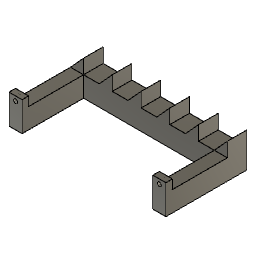
Back_gripper_assembly v17 (Autodesk Fusion 360 archive; units mm, degrees)
design "Wall_reverse"
Autodesk Fusion 360 part; units mm, degrees
sketch "Sketch1" plane through (0, 0, 0) normal (0, 0, 1) x (1, 0, 0)
  line L0 (30, -7.5) -> (-30, -7.5)
  line L1 (-30, -7.5) -> (-30, 7.5)
  line L2 (-30, 7.5) -> (30, 7.5)
  line L3 (30, 7.5) -> (30, -7.5)
  line L4 (30, -7.5) -> (-30, 7.5) construction
  line L5 (-30, -7.5) -> (30, 7.5) construction
  dimension "d1" = 60
  dimension "d2" = 15
  constraint horizontal L0
  constraint perpendicular L0 L1
  constraint parallel L0 L2
  constraint parallel L1 L3
  constraint coincident L4 origin
  constraint coincident L5 origin
  measures "d1" distance of L1.end L2.end
  measures "d2" distance of L0.end L1.end
extrude "Extrude1" add sketch "Sketch1" along normal blind 15.5 makes body 1
sketch "Sketch2" plane through (0, 0, 15.5) normal (0, 0, 1) x (-1, 0, 0)
  line L0 (-30, -7.5) -> (30, -7.5)
  line L1 (30, -7.5) -> (30, 7.5)
  line L2 (30, 7.5) -> (-30, 7.5)
  line L3 (-30, 7.5) -> (-30, -7.5)
  line L4 (-30, -7.5) -> (-15, -7.5)
  line L5 (-15, -7.5) -> (-15, 12.5)
  line L6 (-15, 12.5) -> (-30, 12.5)
  line L7 (-30, 12.5) -> (-30, -7.5)
  dimension "d5" = 15
  dimension "d6" = 20
  constraint horizontal L4
  constraint vertical L5
  constraint horizontal L6
  constraint vertical L7
  constraint coincident L0.start L3.end
  measures "d5" distance of L0.start L4.end
  measures "d6" distance of L0.start L6.end
sketch "Sketch3" plane through (0, -7.5, 0) normal (0, -1, 0) x (1, 0, 0)
  line L0 (-30, 0) -> (30, 0)
  line L1 (30, 0) -> (30, 15.5)
  line L2 (30, 15.5) -> (-30, 15.5)
  line L3 (-30, 15.5) -> (-30, 0)
  line L4 (20, 15.5) -> (30, 15.5)
  line L5 (30, 15.5) -> (30, 0)
  line L6 (30, 0) -> (20, 0)
  line L7 (20, 0) -> (20, 15.5)
  constraint horizontal L4
  constraint vertical L5
  constraint horizontal L6
  constraint vertical L7
  constraint coincident L0.end L1.start
  constraint coincident L1.end L2.start
extrude "Extrude3" add sketch "Sketch3" along normal blind 47 contours L0 L1 L2 L4 L5 L6 L7 bodies 1
sketch "Sketch4" plane through (0, 0, 15.5) normal (0, 0, 1) x (-1, 0, 0)
  line L0 (-30, 54.5) -> (-30, -7.5)
  line L1 (-20, 7.5) -> (-20, 54.5)
  line L2 (-20, 54.5) -> (-30, 54.5)
  line L3 (-20, 54.5) -> (-61.6412, 54.5)
  line L4 (-61.6412, 54.5) -> (-61.6412, 49.5)
  line L5 (-61.6412, 49.5) -> (-20, 49.5)
  line L6 (-20, 49.5) -> (-20, 54.5)
  line L7 (-30, -7.5) -> (30, -7.5)
  line L8 (30, -7.5) -> (30, 7.5)
  line L9 (30, 7.5) -> (-20, 7.5)
  dimension "d11" = 5
  constraint horizontal L3
  constraint vertical L4
  constraint horizontal L5
  constraint vertical L6
  constraint coincident L1.end L2.start
  measures "d11" distance of L1.end L5.end
extrude "Extrude4" add sketch "Sketch4" along normal blind 7 contours L0 L1 L2 L3 L5 L6 bodies 1
mirror "Mirror1" about plane through (-30, -7.5, 0) normal (-1, 0, 0) of bodies 1 merged
sketch "Sketch5" plane through (0, -49.5, 0) normal (0, 1, 0) x (-1, 0, 0)
  line L0 (80, 15.5) -> (90, 15.5)
  line L1 (90, 15.5) -> (90, 22.5)
  line L2 (90, 22.5) -> (80, 22.5)
  line L3 (80, 22.5) -> (80, 15.5)
  circle A0 centre (-25, 19) radius 3
  circle A1 centre (-25, 19) radius 1.5
  circle A2 centre (85, 19) radius 3
  circle A3 centre (85, 19) radius 1.5
  line L4 (-20, 22.5) -> (-30, 22.5)
  line L5 (-20, 15.5) -> (-20, 22.5)
  dimension "d16" = 6
  dimension "d17" = 3
  dimension "d18" = 6
  dimension "d19" = 3
  dimension "d24" = 3.5
  dimension "d25" = 3.5
  dimension "d40" = 5
  dimension "d41" = 5
  constraint concentric A0 A1
  constraint concentric A2 A3
  measures "d16" diameter of A0
  measures "d17" diameter of A1
  measures "d18" diameter of A2
  measures "d19" diameter of A3
  measures "d24" distance of A0.centre L4
  measures "d25" distance of L2 A2.centre
  measures "d40" distance of A0.centre L5
  measures "d41" distance of L1 A2.centre
extrude "Extrude5" cut sketch "Sketch5" against normal blind 15 contours A1 | A3 bodies 1
extrude "Extrude6" cut sketch "Sketch5" against normal blind 2 contours A0 | A2 bodies 1
sketch "Sketch6" plane through (0, 0, 15.5) normal (0, 0, 1) x (-1, 0, 0)
  line L0 (-20, 49.5) -> (-30, 49.5)
  line L1 (-30, 49.5) -> (-30, -7.5)
  line L2 (-30, -7.5) -> (90, -7.5)
  line L3 (90, -7.5) -> (90, 49.5)
  line L4 (90, 49.5) -> (80, 49.5)
  line L5 (80, 49.5) -> (80, 7.5)
  line L6 (80, 7.5) -> (-20, 7.5)
  line L7 (-20, 7.5) -> (-20, 49.5)
  line L8 (-30, -7.5) -> (-20, -7.5)
  line L9 (-20, -7.5) -> (-20, 7.5)
  line L10 (-20, 7.5) -> (-30, 7.5)
  line L11 (-30, 7.5) -> (-30, -7.5)
  constraint horizontal L8
  constraint vertical L9
  constraint horizontal L10
  constraint vertical L11
  constraint coincident L1.end L2.start
  constraint coincident L6.end L7.start
extrude "Extrude7" add sketch "Sketch6" along normal blind 11 contours L1 L2 L8 L9 L10 L11 bodies 1
sketch "Sketch7" plane through (0, -7.5, 0) normal (0, -1, 0) x (1, 0, 0)
  line L0 (20, 15.5) -> (30, 15.5)
  line L1 (30, 15.5) -> (30, 26.5)
  line L2 (30, 26.5) -> (20, 26.5)
  line L3 (20, 26.5) -> (20, 15.5)
  line L4 (20, 26.5) -> (30, 15.5)
  constraint coincident L2.end L3.start
  constraint coincident L0.end L1.start
extrude "Extrude9" cut sketch "Sketch7" against normal through all contours L1 L2 L4 bodies 1
pattern_linear "R-Pattern2" count 6 spacing 22 along (-1, 0, 0) of "Extrude7", "Extrude9"
mirror "Mirror2" about plane through (0, 0, 0) normal (1, 0, 0) of bodies 1 makes body 2
move_body "Move1" bodies 2 to x (1, 0, 0) y (0, 1, 0) z (0, 0, 1) at (-55, 95, 0)
hidden bodies 1

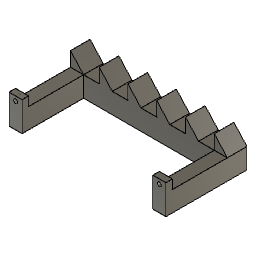
design "Wall"
Autodesk Fusion 360 part; units mm, degrees
sketch "Sketch1" plane through (0, 0, 0) normal (0, 0, 1) x (1, 0, 0)
  line L0 (30, -7.5) -> (-30, -7.5)
  line L1 (-30, -7.5) -> (-30, 7.5)
  line L2 (-30, 7.5) -> (30, 7.5)
  line L3 (30, 7.5) -> (30, -7.5)
  line L4 (30, -7.5) -> (-30, 7.5) construction
  line L5 (-30, -7.5) -> (30, 7.5) construction
  dimension "d1" = 60
  dimension "d2" = 15
  constraint horizontal L0
  constraint perpendicular L0 L1
  constraint parallel L0 L2
  constraint parallel L1 L3
  constraint coincident L4 origin
  constraint coincident L5 origin
  measures "d1" distance of L1.end L2.end
  measures "d2" distance of L0.end L1.end
extrude "Extrude1" add sketch "Sketch1" along normal blind 15.5
sketch "Sketch2" plane through (0, 0, 15.5) normal (0, 0, 1) x (-1, 0, 0)
  line L0 (-30, -7.5) -> (30, -7.5)
  line L1 (30, -7.5) -> (30, 7.5)
  line L2 (30, 7.5) -> (-30, 7.5)
  line L3 (-30, 7.5) -> (-30, -7.5)
  line L4 (-30, -7.5) -> (-15, -7.5)
  line L5 (-15, -7.5) -> (-15, 12.5)
  line L6 (-15, 12.5) -> (-30, 12.5)
  line L7 (-30, 12.5) -> (-30, -7.5)
  dimension "d5" = 15
  dimension "d6" = 20
  constraint horizontal L4
  constraint vertical L5
  constraint horizontal L6
  constraint vertical L7
  constraint coincident L0.start L3.end
  measures "d5" distance of L0.start L4.end
  measures "d6" distance of L0.start L6.end
sketch "Sketch3" plane through (0, -7.5, 0) normal (0, -1, 0) x (1, 0, 0)
  line L0 (-30, 0) -> (30, 0)
  line L1 (30, 0) -> (30, 15.5)
  line L2 (30, 15.5) -> (-30, 15.5)
  line L3 (-30, 15.5) -> (-30, 0)
  line L4 (20, 15.5) -> (30, 15.5)
  line L5 (30, 15.5) -> (30, 0)
  line L6 (30, 0) -> (20, 0)
  line L7 (20, 0) -> (20, 15.5)
  constraint horizontal L4
  constraint vertical L5
  constraint horizontal L6
  constraint vertical L7
  constraint coincident L0.end L1.start
  constraint coincident L1.end L2.start
extrude "Extrude3" add sketch "Sketch3" along normal blind 47 contours L0 L1 L2 L4 L5 L6 L7
sketch "Sketch4" plane through (0, 0, 15.5) normal (0, 0, 1) x (-1, 0, 0)
  line L0 (-30, 54.5) -> (-30, -7.5)
  line L1 (-20, 7.5) -> (-20, 54.5)
  line L2 (-20, 54.5) -> (-30, 54.5)
  line L3 (-20, 54.5) -> (-61.6412, 54.5)
  line L4 (-61.6412, 54.5) -> (-61.6412, 49.5)
  line L5 (-61.6412, 49.5) -> (-20, 49.5)
  line L6 (-20, 49.5) -> (-20, 54.5)
  line L7 (-30, -7.5) -> (30, -7.5)
  line L8 (30, -7.5) -> (30, 7.5)
  line L9 (30, 7.5) -> (-20, 7.5)
  dimension "d11" = 5
  constraint horizontal L3
  constraint vertical L4
  constraint horizontal L5
  constraint vertical L6
  constraint coincident L1.end L2.start
  measures "d11" distance of L1.end L5.end
extrude "Extrude4" add sketch "Sketch4" along normal blind 7 contours L0 L1 L2 L3 L5 L6
mirror "Mirror1" about plane through (-30, -7.5, 0) normal (-1, 0, 0) of bodies 1 merged
sketch "Sketch5" plane through (0, -49.5, 0) normal (0, 1, 0) x (-1, 0, 0)
  line L0 (80, 15.5) -> (90, 15.5)
  line L1 (90, 15.5) -> (90, 22.5)
  line L2 (90, 22.5) -> (80, 22.5)
  line L3 (80, 22.5) -> (80, 15.5)
  circle A0 centre (-25, 19) radius 3
  circle A1 centre (-25, 19) radius 1.5
  circle A2 centre (85, 19) radius 3
  circle A3 centre (85, 19) radius 1.5
  line L4 (-20, 22.5) -> (-30, 22.5)
  line L5 (-20, 15.5) -> (-20, 22.5)
  dimension "d16" = 6
  dimension "d17" = 3
  dimension "d18" = 6
  dimension "d19" = 3
  dimension "d24" = 3.5
  dimension "d25" = 3.5
  dimension "d40" = 5
  dimension "d41" = 5
  constraint concentric A0 A1
  constraint concentric A2 A3
  measures "d16" diameter of A0
  measures "d17" diameter of A1
  measures "d18" diameter of A2
  measures "d19" diameter of A3
  measures "d24" distance of A0.centre L4
  measures "d25" distance of L2 A2.centre
  measures "d40" distance of A0.centre L5
  measures "d41" distance of L1 A2.centre
extrude "Extrude5" cut sketch "Sketch5" against normal blind 15 contours A1 | A3
extrude "Extrude6" cut sketch "Sketch5" against normal blind 2 contours A0 | A2
sketch "Sketch6" plane through (0, 0, 15.5) normal (0, 0, 1) x (-1, 0, 0)
  line L0 (-20, 49.5) -> (-30, 49.5)
  line L1 (-30, 49.5) -> (-30, -7.5)
  line L2 (-30, -7.5) -> (90, -7.5)
  line L3 (90, -7.5) -> (90, 49.5)
  line L4 (90, 49.5) -> (80, 49.5)
  line L5 (80, 49.5) -> (80, 7.5)
  line L6 (80, 7.5) -> (-20, 7.5)
  line L7 (-20, 7.5) -> (-20, 49.5)
  line L8 (-30, -7.5) -> (-20, -7.5)
  line L9 (-20, -7.5) -> (-20, 7.5)
  line L10 (-20, 7.5) -> (-30, 7.5)
  line L11 (-30, 7.5) -> (-30, -7.5)
  constraint horizontal L8
  constraint vertical L9
  constraint horizontal L10
  constraint vertical L11
  constraint coincident L1.end L2.start
  constraint coincident L6.end L7.start
extrude "Extrude7" add sketch "Sketch6" along normal blind 11 contours L1 L2 L8 L9 L10 L11
sketch "Sketch7" plane through (0, -7.5, 0) normal (0, -1, 0) x (1, 0, 0)
  line L0 (20, 15.5) -> (30, 15.5)
  line L1 (30, 15.5) -> (30, 26.5)
  line L2 (30, 26.5) -> (20, 26.5)
  line L3 (20, 26.5) -> (20, 15.5)
  line L4 (20, 26.5) -> (30, 15.5)
  constraint coincident L2.end L3.start
  constraint coincident L0.end L1.start
extrude "Extrude9" cut sketch "Sketch7" against normal through all contours L1 L2 L4
pattern_linear "R-Pattern2" count 6 spacing 22 along (-1, 0, 0) of "Extrude7", "Extrude9"

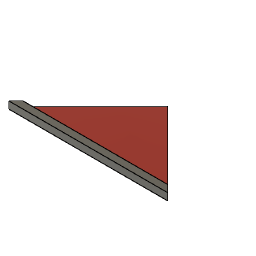
design "New_sqaure"
Autodesk Fusion 360 part; units mm, degrees
sketch "Sketch1" plane through (0, 0, 0) normal (0, 0, 1) x (1, 0, 0)
  line L0 (0, 0) -> (0, 112)
  line L1 (0, 0) -> (112, 0)
  line L2 (0, 112) -> (112, 0)
  line L3 (0, 112) -> (-112, 0)
  line L4 (0, 0) -> (-112, 0)
  dimension "d3" = 112
  dimension "d4" = 112
  dimension "d5" = 158.3919
  constraint coincident L0.start L1.start
  constraint vertical L0
  constraint perpendicular L0 L1
  constraint symmetric L2.start L0 L3.start
  constraint symmetric L0 L1.start L4.start
  constraint symmetric L0 L1.end L3.end
  measures "d3" distance of L0.start L0.end
  measures "d4" distance of L0.start L1.end
  measures "d5" distance of L0.end L1.end
extrude "Extrude1" add sketch "Sketch1" along normal blind 3
sketch "Sketch2" plane through (0, 0, 0) normal (0, 0, -1) x (1, 0, 0)
  line L0 (-112, 0) -> (0, -112)
  line L1 (0, -112) -> (112, 0)
  line L2 (112, 0) -> (-112, 0)
  line L3 (0, 0) -> (0, -10) construction
  line L4 (0, -10) -> (115, -10)
  line L5 (115, -10) -> (-102, -10)
  dimension "d8" = 10
  constraint coincident L3.start origin
  constraint perpendicular L2 L3
  constraint perpendicular L3 L4
  constraint coincident L0 L5.end
  constraint perpendicular L3 L5
  measures "d8" distance of L3.start L3.end
sketch "Sketch3" plane through (0, 0, 3) normal (0, 0, 1) x (-1, 0, 0)
  line L0 (0, -112) -> (112, 0)
  line L1 (112, 0) -> (-112, 0)
  line L2 (-112, 0) -> (0, -112)
  line L3 (0, 0) -> (0, -10) construction
  line L4 (0, -10) -> (115, -10)
  line L5 (115, -10) -> (-102, -10)
  dimension "d11" = 10
  constraint coincident L3.start origin
  constraint perpendicular L1 L3
  constraint perpendicular L3 L4
  constraint coincident L2 L5.end
  constraint perpendicular L3 L5
  measures "d11" distance of L3.start L3.end
extrude "Extrude3" add sketch "Sketch3" along normal blind 7 contours L0 L1 L2 L4 L5
sketch "Sketch4" plane through (0, 0, 0) normal (0, -1, 0) x (1, 0, 0)
  line L0 (112, 0) -> (112, 10)
  line L1 (112, 10) -> (-112, 10)
  line L2 (-112, 10) -> (-112, 0)
  line L3 (0, 0) -> (-112, 0)
  line L4 (0, 0) -> (112, 0)
  line L5 (-112, 0) -> (112, 0)
  constraint coincident L3.start L4.start
  constraint coincident L2 L3.end
  constraint perpendicular L2 L3
  constraint coincident L0 L4.end
  constraint perpendicular L0 L4
extrude "Extrude4" [suppressed]
equation "Height_lenght = 112 mm"
equation "Sqaure_lenght = sqrt(2) * Height_lenght"
equation "d3 = Height_lenght"
equation "d4 = Height_lenght"
equation "d5 = Sqaure_lenght"

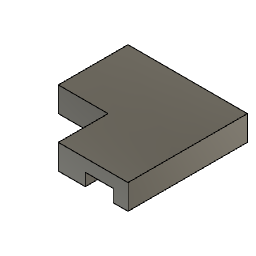
design "corner"
Autodesk Fusion 360 part; units mm, degrees
sketch "Sketch1" plane through (0, 0, 0) normal (0, 0, 1) x (1, 0, 0)
  circle A0 centre (0, 0) radius 22
  circle A1 centre (0, 0) radius 11
  line L0 (0, 0) -> (0, 20)
  line L1 (0, 0) -> (26, 0)
  line L2 (0, 0) -> (28, 0)
  line L3 (28, 0) -> (28, 28)
  line L4 (28, 28) -> (0, 28)
  line L5 (0, 28) -> (0, 0)
  line L6 (0, 11) -> (0, 22) construction
  line L7 (11, 0) -> (13, 0) construction
  arc A2 (11, 0) -> (0, 11) centre (0.4983, 0.4983) ccw construction
  dimension "d1" = 44
  dimension "d2" = 22
  constraint coincident A0.centre A1.centre
  constraint concentric A0 A1
  constraint vertical L0
  constraint perpendicular L0 L1
  constraint horizontal L2
  constraint vertical L3
  constraint horizontal L4
  constraint vertical L5
  constraint coincident A1 L6.start
  constraint coincident L0 L6.start
  constraint coincident L0 L6.end
  constraint coincident A0 L6.end
  constraint coincident A1 L7.start
  constraint coincident L1 L7.start
  constraint midpoint L1 L7.end
  constraint perpendicular L6 L7
  measures "d1" diameter of A0
  measures "d2" diameter of A1
extrude "Extrude1" add sketch "Sketch1" along normal blind 10 contours A0 A1 L0 L1 L2 L5 | A0 L1 L2 L3 L4 L5 | A1 L0 L1 L2 L5 picked at (3.0991, 17.2211) picked at (3.5055, 6.4199)
extrude "Extrude2" cut sketch "Sketch1" along normal blind 5 contours A0 A1 L0 L1 L2 L5 picked at (3.0991, 17.2211)
extrude "Extrude4" add 1 faces at (0, 3.6667, 5) along direction (-1, 0, 0) blind 20
sketch "Sketch5" plane through (0, 0, 0) normal (0, 1, 0) x (1, 0, 0)
  line L0 (28, 0) -> (0, 0)
  line L1 (0, 0) -> (0, -10)
  line L2 (0, -10) -> (28, -10)
  line L3 (28, -10) -> (28, 0)
  line L4 (22, -5) -> (10.8427, -5)
  line L5 (10.8427, -5) -> (10.8427, 0)
  line L6 (10.8427, 0) -> (22, 0)
  line L7 (22, 0) -> (22, -5)
  constraint horizontal L0
  constraint vertical L1
  constraint horizontal L2
  constraint vertical L3
  constraint horizontal L4
  constraint vertical L5
  constraint horizontal L6
  constraint vertical L7
  constraint coincident L0 L5.end
extrude "Extrude5" add sketch "Sketch5" against normal blind 20 contours L0 L1 L2 L3 L4 L5 L7
sketch "Sketch6" plane through (0, 0, 0) normal (0, 0, -1) x (1, 0, 0)
  arc A0 (0, -11) -> (11, 0) centre (0, 0) ccw
  line L0 (11, 0) -> (10.8427, 0)
  line L1 (10.8427, 0) -> (10.8427, 20)
  line L2 (10.8427, 20) -> (0, 20)
  line L3 (0, 20) -> (0, 0)
  line L4 (0, 0) -> (-20, 0)
  line L5 (-20, 0) -> (-20, -11)
  line L6 (-20, -11) -> (0, -11)
  line L7 (10.8427, 0) -> (0, 0)
  line L8 (0, 0) -> (0, -11)
  circle A1 centre (0, 0) radius 5
  dimension "d18" = 10
  constraint coincident L0.end L1.start
  constraint coincident A0.centre L3.end
  constraint coincident A0.start L6.end
  measures "d18" diameter of A1
extrude "Extrude6" cut sketch "Sketch6" against normal blind 5 contours A0 L0 L7 L8 A1
fillet "Fillet1" radius 5 2 edges at (10.8427, 0, 2.5) (0, 11, 2.5)
